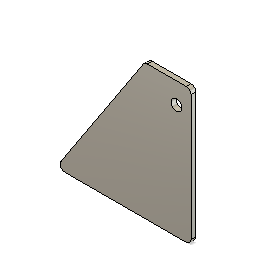
Test+intake+shooter+and+intake (Autodesk Fusion 360 design; units mm, degrees)
Autodesk Fusion 360 part; units mm, degrees
sketch "Sketch1" plane through (0, 0, 0) normal (0, 0, 1) x (1, 0, 0)
  line L0 (0, 0) -> (355.6, 0)
  line L1 (355.6, 0) -> (355.6, 355.6)
  line L2 (355.6, 355.6) -> (233.4623, 355.6)
  circle A0 centre (317.5, 300.4312) radius 14.2748
  line L3 (233.4623, 355.6) -> (0, 0)
  dimension "d1" = 355.6
  dimension "d3" = 28.5496
  dimension "d4" = 300.4312
  dimension "d5" = 38.1
  constraint horizontal L0
  constraint vertical L1
  constraint horizontal L2
  constraint coincident L0.start L3.end
  measures "d1" distance of L0.start L0.end
  measures "d3" diameter of A0
  measures "d4" distance of L0 A0.centre
  measures "d5" distance of L1 A0.centre
extrude "Extrude1" add sketch "Sketch1" along normal blind 12.7
fillet "Fillet1" radius 12.7 4 edges at (355.6, 355.6, 6.35) (233.4623, 355.6, 6.35) (355.6, 0, 6.35) (0, 0, 6.35)
